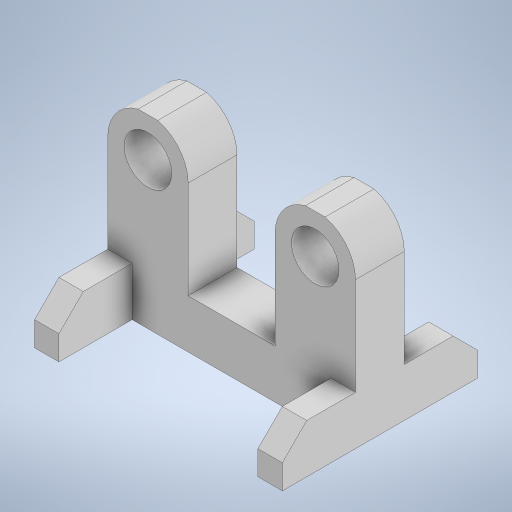
# Autodesk Inventor part: Guide Rod Support
Saved by Autodesk Inventor 2024 (Build 280153000, 153)
## iProperties
Manager: Scott J. Bricker
Company: University of California - Davis
Created: 2024-11-21
Part Number: Guide Rod Support
Project: Firgelli Motorized Linear Stage
Material: Generic
Document SubType Name: Modeling
Designer: Scott J. Bricker
Engineer: Scott J. Bricker
Density: 1 g/cm^3
Appearance: Default
Title: Guide Rod Support
Subject: Firgelli Motorized Linear Stage
Author: Scott J. Bricker
Revision Number: 1.1 P3
Autodesk Inventor part; units mm, degrees
ref_plane "YZ Plane" through (0, 0, 0) normal (1, 0, 0) x (0, 1, 0)
ref_plane "XZ Plane" through (0, 0, 0) normal (0, 1, 0) x (-1, 0, 0)
sketch "Sketch1" plane through (0, 0, 0) normal (0, 0, 1) x (1, 0, 0)
  line L0 (0, 0) -> (50.8, 0)
  line L1 (50.8, 0) -> (50.8, 10)
  line L2 (0, 10) -> (0, 0)
  circle A0 centre (8.25, 30) radius 4.875
  arc A1 (16.5, 30) -> (0, 30) centre (8.25, 30) ccw
  line L3 (25.4, -5.1734) -> (25.4, 32.937)
  line L4 (0, 30) -> (0, 10)
  line L5 (16.5, 30) -> (16.5, 10)
  line L6 (50.8, 10) -> (16.5, 10)
  line L7 (0, 10) -> (0, 10)
  circle A2 centre (42.55, 30) radius 4.875
  arc A3 (50.8, 30) -> (34.3, 30) centre (42.55, 30) ccw
  line L8 (50.8, 30) -> (50.8, 10)
  line L9 (34.3, 30) -> (34.3, 10)
  line L10 (-14.5687, 38) -> (58.8919, 38)
  line L11 (58.8919, 38) -> (58.8919, 91.2703)
  line L12 (58.8919, 91.2703) -> (-14.5687, 91.2703)
  line L13 (-14.5687, 91.2703) -> (-14.5687, 38)
  point P0 (25.4, 0)
  point P1 (34.3, 10)
  point P2 (44.5656, 38)
  point P3 (40.5344, 38)
  point P4 (10.2656, 38)
  point P5 (6.2344, 38)
  dimension "d0" = 0
  dimension "d1" = 50.8
  dimension "d2" = 8.25
  dimension "d3" = 9.75
  dimension "d4" = 16.5
  dimension "d7" = 10
  dimension "d8" = 0
  dimension "d19" = 20
  dimension "d21" = 28
  constraints: 28 end point, 6 perpendicular, 6 symmetric about line, 5 parallel, 4 centre point, 4 point on circle, 2 coincident, 2 horizontal, 2 tangent, 1 midpoint, 1 vertical, 2 other
  measures "d0" distance from line of point (25.4, 0) L3
  measures "d1" distance of L0.start L0.end
  measures "d2" distance from line of L2 A0.centre
  measures "d3" diameter of A0
  measures "d4" diameter of A1
  measures "d7" distance between parallel lines of L0 L6
  measures "d8" distance between parallel lines of L6 L7
  measures "d19" distance from line of L6 A1.centre
  measures "d21" distance between parallel lines of L6 L10
extrude "Extrusion1" add sketch "Sketch1" along normal blind 10 contours L2 L4 A1 L10 L5 L6 L3 L0 | L3 L6 L1 L0 | L6 L9 A3 L10 L8
ref_plane "Work Plane1" through (0, 0, 5) normal (0, 0, 1) x (1, 0, 0)
sketch "Sketch2" plane through (0, 0, 5) normal (0, 0, 1) x (1, 0, 0)
  line L0 (0, 0) -> (50.8, 0) projected
  line L1 (50.8, 0) -> (50.8, 30) projected
  arc A0 (50.8, 30) -> (44.5656, 38) centre (42.55, 30) ccw projected
  line L2 (34.3, 30) -> (34.3, 10) projected
  line L3 (34.3, 10) -> (16.5, 10) projected
  line L4 (16.5, 10) -> (16.5, 30) projected
  arc A1 (16.5, 30) -> (10.2656, 38) centre (8.25, 30) ccw projected
  line L5 (0, 30) -> (0, 0) projected
  circle A2 centre (42.55, 30) radius 4.875 projected
  circle A3 centre (8.25, 30) radius 4.875 projected
  line L6 (0, 0) -> (5, 0)
  line L7 (5, 0) -> (5, 10)
  line L8 (5, 10) -> (0, 10)
  line L9 (0, 10) -> (0, 0)
  line L10 (50.8, 0) -> (45.8, 0)
  line L11 (45.8, 0) -> (45.8, 10)
  line L12 (45.8, 10) -> (50.8, 10)
  line L13 (50.8, 10) -> (50.8, 0)
  line L14 (44.5656, 38) -> (40.5344, 38) projected
  arc A4 (40.5344, 38) -> (34.3, 30) centre (42.55, 30) ccw projected
  line L15 (10.2656, 38) -> (6.2344, 38) projected
  arc A5 (6.2344, 38) -> (0, 30) centre (8.25, 30) ccw projected
  dimension "d10" = 5
  dimension "d11" = 5
  dimension "d12" = 10
  dimension "d13" = 10
  constraints: 16 end point, 4 parallel, 2 horizontal, 2 perpendicular
  measures "d10" distance of L7.end L8.end
  measures "d11" distance of L11.end L12.end
  measures "d12" distance of L6.end L7.end
  measures "d13" distance of L10.end L11.end
extrude "Extrusion2" add sketch "Sketch2" along normal mid plane 40 contours L5 L8 L7 L0 | L11 L12 L1 L0
chamfer "Chamfer1" distance 5 angle 45 4 edges at (2.5, 10, 25) (48.3, 10, 25) (48.3, 10, -15) (2.5, 10, -15)
equation "\"d2\" = 0.5 * Platform_GuideRod_OD"
equation "\"d4\" = Platform_GuideRod_OD"
equation "\"d7\" = Thick_Wall"
equation "\"d21\" = Sliding_Clearance + Actuator_Housing_W"
equation "\"d5\" = Thick_Wall"
equation "\"d11\" = d10"
equation "\"d12\" = Thick_Wall"
equation "\"d13\" = d12"
equation "\"d16\" = 0.5 * Thick_Wall"
equation "\"Platform_Width\" = 50.8"
equation "\"Platform_Length\" = 245"
equation "\"Guide_Hole_Offset\" = 13.51"
equation "\"Guide_Rod_Diameter\" = 6"
equation "\"Guide_Rod_Length\" = 304.8"
equation "\"Thin_Wall\" = 5"
equation "\"Thick_Wall\" = 10"
equation "\"Tabletop_Hole_Spacing\" = 25.4"
equation "\"Tabletop_Hole_Diameter\" = 6.35"
equation "\"Platform_Hole_Spacing\" = 25.4"
equation "\"Platform_Hole_Diameter\" = 6.35"
equation "\"Actuator_Housing_W\" = 26"
equation "\"Sliding_Clearance\" = 2"
equation "\"Platform_GuideRod_OD\" = 16.5"
equation "\"d9\" = -0.5 * Thick_Wall"
body "Solid1"
